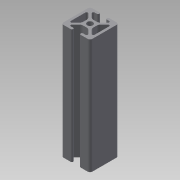
# Autodesk Inventor part: 25-2504
Saved by Autodesk Inventor 2013 (Build 170138000, 138)
## iProperties
Created: 2014-04-23
Part Number: 25-2504
Material: Generic
Document SubType Name: Modeling
Designer: Ross Bowman
Density: 1 g/cm^3
Engineer: Ross Bowman
Catalog Web Link: 8020.net
Vendor: 80/20 Inc.
Company: 80/20 Inc.
Author: Ross Bowman
Keywords: 80/20 , 8020 , T-Slot , Extrusion
Material: 6105-T5 Aluminum
Autodesk Inventor part; units mm, degrees
ref_plane "YZ Plane" through (0, 0, 0) normal (1, 0, 0) x (0, 1, 0)
ref_plane "XZ Plane" through (0, 0, 0) normal (0, 1, 0) x (-1, 0, 0)
ref_plane "XY Plane" through (0, 0, 0) normal (0, 0, 1) x (1, 0, 0)
sketch "Sketch1" plane through (0, 0, 0) normal (0, 0, 1) x (1, 0, 0)
  arc A0 (-10.36, -6.4282) -> (-8.6498, -7.1366) centre (-9.3582, -6.4282) ccw
  line L0 (-10.36, 6.4282) -> (-10.36, -6.4282)
  arc A1 (-8.6498, 7.1366) -> (-10.36, 6.4282) centre (-9.3582, 6.4282) ccw
  line L1 (-5.3093, 3.7961) -> (-8.6498, 7.1366)
  arc A2 (-4.38, 1.5525) -> (-5.3093, 3.7961) centre (-7.553, 1.5525) ccw
  line L2 (-4.38, -1.5525) -> (-4.38, 1.5525)
  arc A3 (-5.3093, -3.7961) -> (-4.38, -1.5525) centre (-7.553, -1.5525) ccw
  line L3 (-8.6498, -7.1366) -> (-5.3093, -3.7961)
  arc A4 (8.6498, -7.1366) -> (10.36, -6.4282) centre (9.3582, -6.4282) ccw
  line L4 (5.3093, -3.7961) -> (8.6498, -7.1366)
  arc A5 (4.38, -1.5525) -> (5.3093, -3.7961) centre (7.553, -1.5525) ccw
  line L5 (4.38, 1.5525) -> (4.38, -1.5525)
  arc A6 (5.3093, 3.7961) -> (4.38, 1.5525) centre (7.553, 1.5525) ccw
  line L6 (8.6498, 7.1366) -> (5.3093, 3.7961)
  arc A7 (10.36, 6.4282) -> (8.6498, 7.1366) centre (9.3582, 6.4282) ccw
  line L7 (10.36, -6.4282) -> (10.36, 6.4282)
  circle A8 centre (0, 0) radius 2.5
  line L8 (-10.5183, -12.5) -> (-4.32, -12.5)
  arc A9 (-4.32, -12.5) -> (-4.32, -10.36) centre (-4.32, -11.43) ccw
  line L9 (-4.32, -10.36) -> (-6.4282, -10.36)
  arc A10 (-7.1366, -8.6498) -> (-6.4282, -10.36) centre (-6.4282, -9.3582) ccw
  line L10 (-7.1366, -8.6498) -> (-3.7961, -5.3093)
  arc A11 (-1.5525, -4.38) -> (-3.7961, -5.3093) centre (-1.5525, -7.553) ccw
  line L11 (-1.5525, -4.38) -> (1.5525, -4.38)
  arc A12 (3.7961, -5.3093) -> (1.5525, -4.38) centre (1.5525, -7.553) ccw
  line L12 (3.7961, -5.3093) -> (7.1366, -8.6498)
  arc A13 (6.4282, -10.36) -> (7.1366, -8.6498) centre (6.4282, -9.3582) ccw
  line L13 (6.4282, -10.36) -> (4.32, -10.36)
  arc A14 (4.32, -10.36) -> (4.32, -12.5) centre (4.32, -11.43) ccw
  line L14 (4.32, -12.5) -> (10.5183, -12.5)
  arc A15 (10.5183, -12.5) -> (12.5, -10.5183) centre (10.5183, -10.5183) ccw
  line L15 (12.5, -10.5183) -> (12.5, 10.5183)
  arc A16 (12.5, 10.5183) -> (10.5183, 12.5) centre (10.5183, 10.5183) ccw
  line L16 (10.5183, 12.5) -> (4.32, 12.5)
  arc A17 (4.32, 12.5) -> (4.32, 10.36) centre (4.32, 11.43) ccw
  line L17 (4.32, 10.36) -> (6.4282, 10.36)
  arc A18 (7.1366, 8.6498) -> (6.4282, 10.36) centre (6.4282, 9.3582) ccw
  line L18 (7.1366, 8.6498) -> (3.7961, 5.3093)
  arc A19 (1.5525, 4.38) -> (3.7961, 5.3093) centre (1.5525, 7.553) ccw
  line L19 (1.5525, 4.38) -> (-1.5525, 4.38)
  arc A20 (-3.7961, 5.3093) -> (-1.5525, 4.38) centre (-1.5525, 7.553) ccw
  line L20 (-3.7961, 5.3093) -> (-7.1366, 8.6498)
  arc A21 (-6.4282, 10.36) -> (-7.1366, 8.6498) centre (-6.4282, 9.3582) ccw
  line L21 (-6.4282, 10.36) -> (-4.32, 10.36)
  arc A22 (-4.32, 10.36) -> (-4.32, 12.5) centre (-4.32, 11.43) ccw
  line L22 (-4.32, 12.5) -> (-10.5183, 12.5)
  arc A23 (-10.5183, 12.5) -> (-12.5, 10.5183) centre (-10.5183, 10.5183) ccw
  line L23 (-12.5, 10.5183) -> (-12.5, -10.5183)
  arc A24 (-12.5, -10.5183) -> (-10.5183, -12.5) centre (-10.5183, -10.5183) ccw
  constraints: 48 end point, 48 point on circle, 25 centre point
extrude "Extrusion1" add sketch "Sketch1" against normal blind 100
body "Solid1"
